Autodesk Inventor part; units mm, degrees
(part 2 of 3)
sketch "Skizze14" plane through (-77, -91.5, 192.5) normal (0.7071, 0, 0.7071) x (0.7071, 0, -0.7071)
  line L0 (0.4493, 19.9089) -> (5.7022, 19.9089) construction
  line L1 (5.7022, 19.9089) -> (5.7022, 29.9599) construction
  line L2 (5.7022, 29.9599) -> (0.4493, 29.9599) construction
  line L3 (0.4493, 29.9599) -> (0.4493, 19.9089) construction
  line L4 (0.4923, 49.8867) -> (5.7451, 49.8867) construction
  line L5 (5.7451, 49.8867) -> (5.7451, 46.2392) construction
  line L6 (5.7451, 46.2392) -> (0.4923, 46.2392) construction
  line L7 (0.4923, 46.2392) -> (0.4923, 49.8867) construction
  line L8 (0.1277, 60.4817) -> (5.3805, 60.4817) construction
  line L9 (5.3805, 60.4817) -> (5.3805, 56.8342) construction
  line L10 (5.3805, 56.8342) -> (0.1277, 56.8342) construction
  line L11 (0.1277, 56.8342) -> (0.1277, 60.4817) construction
  line L12 (0.177, 70.1367) -> (5.4298, 70.1367) construction
  line L13 (5.4298, 70.1367) -> (5.4298, 66.4892) construction
  line L14 (5.4298, 66.4892) -> (0.177, 66.4892) construction
  line L15 (0.177, 66.4892) -> (0.177, 70.1367) construction
  line L16 (0.177, 80.1367) -> (5.4298, 80.1367) construction
  line L17 (5.4298, 80.1367) -> (5.4298, 76.4892) construction
  line L18 (5.4298, 76.4892) -> (0.177, 76.4892) construction
  line L19 (0.177, 76.4892) -> (0.177, 80.1367) construction
  line L20 (0.177, 90.1367) -> (5.4298, 90.1367) construction
  line L21 (5.4298, 90.1367) -> (5.4298, 86.4892) construction
  line L22 (5.4298, 86.4892) -> (0.177, 86.4892) construction
  line L23 (0.177, 86.4892) -> (0.177, 90.1367) construction
  line L24 (0.177, 100.1367) -> (5.4298, 100.1367) construction
  line L25 (5.4298, 100.1367) -> (5.4298, 96.4892) construction
  line L26 (5.4298, 96.4892) -> (0.177, 96.4892) construction
  line L27 (0.177, 96.4892) -> (0.177, 100.1367) construction
  line L28 (0.177, 110.1367) -> (5.4298, 110.1367) construction
  line L29 (5.4298, 110.1367) -> (5.4298, 106.4892) construction
  line L30 (5.4298, 106.4892) -> (0.177, 106.4892) construction
  line L31 (0.177, 106.4892) -> (0.177, 110.1367) construction
  line L32 (-0.2126, 120.6134) -> (5.0402, 120.6134) construction
  line L33 (5.0402, 120.6134) -> (5.0402, 116.9659) construction
  line L34 (5.0402, 116.9659) -> (-0.2126, 116.9659) construction
  line L35 (-0.2126, 116.9659) -> (-0.2126, 120.6134) construction
  line L36 (-0.2161, 130.1063) -> (5.0368, 130.1063) construction
  line L37 (5.0368, 130.1063) -> (5.0368, 126.4588) construction
  line L38 (5.0368, 126.4588) -> (-0.2161, 126.4588) construction
  line L39 (-0.2161, 126.4588) -> (-0.2161, 130.1063) construction
  line L40 (-0.2978, 140.1) -> (4.9551, 140.1) construction
  line L41 (4.9551, 140.1) -> (4.9551, 136.4525) construction
  line L42 (4.9551, 136.4525) -> (-0.2978, 136.4525) construction
  line L43 (-0.2978, 136.4525) -> (-0.2978, 140.1) construction
  line L44 (-0.3019, 150.1519) -> (4.9509, 150.1519) construction
  line L45 (4.9509, 150.1519) -> (4.9509, 146.5044) construction
  line L46 (4.9509, 146.5044) -> (-0.3019, 146.5044) construction
  line L47 (-0.3019, 146.5044) -> (-0.3019, 150.1519) construction
  line L48 (-0.2744, 160.1018) -> (4.9784, 160.1018) construction
  line L49 (4.9784, 160.1018) -> (4.9784, 156.4543) construction
  line L50 (4.9784, 156.4543) -> (-0.2744, 156.4543) construction
  line L51 (-0.2744, 156.4543) -> (-0.2744, 160.1018) construction
  line L52 (-0.539, 170.1317) -> (4.1973, 170.1317) construction
  line L53 (4.1973, 170.1317) -> (4.1973, 166.4842) construction
  line L54 (4.1973, 166.4842) -> (-0.539, 166.4842) construction
  line L55 (-0.539, 166.4842) -> (-0.539, 170.1317) construction
  line L56 (0.5265, 39.54) -> (5.7793, 39.54) construction
  line L57 (5.7793, 39.54) -> (5.7793, 35.8925) construction
  line L58 (5.7793, 35.8925) -> (0.5265, 35.8925) construction
  line L59 (0.5265, 35.8925) -> (0.5265, 39.54) construction
  line L60 (8.4853, 5) -> (8.4853, 29.5) projected
  line L61 (12.1672, 16.75) -> (4.8034, 16.75)
  line L62 (4.8034, 16.75) -> (4.8034, 17.75)
  line L63 (4.8034, 17.75) -> (12.1672, 17.75)
  line L64 (12.1672, 17.75) -> (12.1672, 16.75)
  line L65 (12.1672, 16.75) -> (4.8034, 17.75) construction
  line L66 (4.8034, 16.75) -> (12.1672, 17.75) construction
  line L67 (7.3114, 17.75) -> (7.3114, 16.75)
  line L68 (2.9776, 164.5202) -> (0.2945, 164.5202)
  line L69 (0.2945, 164.5202) -> (0.2945, 165.0818)
  line L70 (0.2945, 165.0818) -> (1.2928, 165.0818)
  line L71 (1.2928, 165.0818) -> (1.2928, 168.7678)
  line L72 (1.2928, 168.7678) -> (0.2945, 168.7678)
  line L73 (0.2945, 168.7678) -> (0.2945, 169.2715)
  spline S0 degree 2 poles (0.2945, 169.2715) (0.8605, 169.2715) (1.3954, 169.5924) (1.431, 170.0381) knots 0 0 0 1 2 2 2
  line L74 (1.431, 170.0381) -> (2.0015, 170.0381)
  line L75 (2.0015, 170.0381) -> (2.0015, 165.0818)
  line L76 (2.0015, 165.0818) -> (2.9776, 165.0818)
  line L77 (2.9776, 165.0818) -> (2.9776, 164.5202)
  spline S1 degree 2 poles (7.4659, 166.3031) (7.4659, 165.8796) (7.1851, 165.1621) (6.9488, 164.9214) knots 0 0 0 1 2 2 2
  spline S2 degree 2 poles (6.9488, 164.9214) (6.7037, 164.6673) (6.0886, 164.4044) (5.7187, 164.4044) knots 0 0 0 1 2 2 2
  spline S3 degree 2 poles (5.7187, 164.4044) (5.3488, 164.4044) (4.7381, 164.6539) (4.5064, 164.9035) knots 0 0 0 1 2 2 2
  spline S4 degree 2 poles (4.5064, 164.9035) (4.2211, 165.2022) (3.9002, 166.205) (3.9002, 166.936) knots 0 0 0 1 2 2 2
  spline S5 degree 2 poles (3.9002, 166.936) (3.9002, 167.6535) (4.1944, 168.8079) (4.5019, 169.2358) knots 0 0 0 1 2 2 2
  spline S6 degree 2 poles (4.5019, 169.2358) (4.8005, 169.6548) (5.7454, 170.1227) (6.365, 170.1227) knots 0 0 0 1 2 2 2
  spline S7 degree 2 poles (6.365, 170.1227) (6.5477, 170.1227) (6.8686, 170.0871) (6.989, 170.047) knots 0 0 0 1 2 2 2
  line L78 (6.989, 170.047) -> (6.989, 169.3383)
  line L79 (6.989, 169.3383) -> (6.9578, 169.3383)
  spline S8 degree 2 poles (6.9578, 169.3383) (6.8552, 169.3918) (6.4808, 169.4854) (6.2669, 169.4854) knots 0 0 0 1 2 2 2
  spline S9 degree 2 poles (6.2669, 169.4854) (5.5805, 169.4854) (4.7381, 168.5583) (4.6579, 167.6491) knots 0 0 0 1 2 2 2
  spline S10 degree 2 poles (4.6579, 167.6491) (4.9209, 167.8318) (5.4736, 168.0324) (5.8034, 168.0324) knots 0 0 0 1 2 2 2
  spline S11 degree 2 poles (5.8034, 168.0324) (6.1243, 168.0324) (6.6056, 167.9031) (6.8686, 167.707) knots 0 0 0 1 2 2 2
  spline S12 degree 2 poles (6.8686, 167.707) (7.1717, 167.4797) (7.4659, 166.7755) (7.4659, 166.3031) knots 0 0 0 1 2 2 2
  spline S13 degree 2 poles (6.7171, 166.2719) (6.7171, 166.6106) (6.5388, 167.0697) (6.3427, 167.2301) knots 0 0 0 1 2 2 2
  spline S14 degree 2 poles (6.3427, 167.2301) (6.1956, 167.346) (5.8301, 167.4218) (5.6385, 167.4218) knots 0 0 0 1 2 2 2
  spline S15 degree 2 poles (5.6385, 167.4218) (5.38, 167.4218) (4.8941, 167.2658) (4.6579, 167.1187) knots 0 0 0 1 2 2 2
  spline S16 degree 2 poles (4.6579, 167.1187) (4.6535, 167.0385) (4.6445, 166.8869) (4.6445, 166.771) knots 0 0 0 1 2 2 2
  spline S17 degree 2 poles (4.6445, 166.771) (4.6445, 166.2005) (4.8674, 165.5008) (5.0368, 165.318) knots 0 0 0 1 2 2 2
  spline S18 degree 2 poles (5.0368, 165.318) (5.1928, 165.1442) (5.5315, 165.0061) (5.7231, 165.0061) knots 0 0 0 1 2 2 2
  spline S19 degree 2 poles (5.7231, 165.0061) (6.1689, 165.0061) (6.7171, 165.639) (6.7171, 166.2719) knots 0 0 0 1 2 2 2
  spline S20 degree 2 poles (11.5396, 167.2702) (11.5396, 165.7905) (10.6794, 164.4044) (9.7835, 164.4044) knots 0 0 0 1 2 2 2
  spline S21 degree 2 poles (9.7835, 164.4044) (8.8743, 164.4044) (8.023, 165.8172) (8.023, 167.2658) knots 0 0 0 1 2 2 2
  spline S22 degree 2 poles (8.023, 167.2658) (8.023, 168.7544) (8.8832, 170.1317) (9.7835, 170.1317) knots 0 0 0 1 2 2 2
  spline S23 degree 2 poles (9.7835, 170.1317) (10.6883, 170.1317) (11.5396, 168.7054) (11.5396, 167.2702) knots 0 0 0 1 2 2 2
  spline S24 degree 2 poles (10.5947, 165.5944) (10.7017, 165.8663) (10.7908, 166.7042) (10.7908, 167.2702) knots 0 0 0 1 2 2 2
  spline S25 degree 2 poles (10.7908, 167.2702) (10.7908, 167.8363) (10.7017, 168.6697) (10.5902, 168.9505) knots 0 0 0 1 2 2 2
  spline S26 degree 2 poles (10.5902, 168.9505) (10.4788, 169.2313) (10.0911, 169.521) (9.7835, 169.521) knots 0 0 0 1 2 2 2
  spline S27 degree 2 poles (9.7835, 169.521) (9.476, 169.521) (9.0793, 169.2313) (8.9634, 168.9416) knots 0 0 0 1 2 2 2
  spline S28 degree 2 poles (8.9634, 168.9416) (8.852, 168.6608) (8.7718, 167.8051) (8.7718, 167.2658) knots 0 0 0 1 2 2 2
  spline S29 degree 2 poles (8.7718, 167.2658) (8.7718, 166.6864) (8.8431, 165.9108) (8.959, 165.6078) knots 0 0 0 1 2 2 2
  spline S30 degree 2 poles (8.959, 165.6078) (9.0659, 165.3225) (9.4626, 165.015) (9.7835, 165.015) knots 0 0 0 1 2 2 2
  spline S31 degree 2 poles (9.7835, 165.015) (10.0866, 165.015) (10.4833, 165.3047) (10.5947, 165.5944) knots 0 0 0 1 2 2 2
  line L80 (3.2422, 154.4903) -> (0.559, 154.4903)
  line L81 (0.559, 154.4903) -> (0.559, 155.0519)
  line L82 (0.559, 155.0519) -> (1.5574, 155.0519)
  line L83 (1.5574, 155.0519) -> (1.5574, 158.7379)
  line L84 (1.5574, 158.7379) -> (0.559, 158.7379)
  line L85 (0.559, 158.7379) -> (0.559, 159.2416)
  spline S32 degree 2 poles (0.559, 159.2416) (1.1251, 159.2416) (1.6599, 159.5625) (1.6956, 160.0082) knots 0 0 0 1 2 2 2
  line L86 (1.6956, 160.0082) -> (2.2661, 160.0082)
  line L87 (2.2661, 160.0082) -> (2.2661, 155.0519)
  line L88 (2.2661, 155.0519) -> (3.2422, 155.0519)
  line L89 (3.2422, 155.0519) -> (3.2422, 154.4903)
  spline S33 degree 2 poles (7.5878, 156.2375) (7.5878, 155.8408) (7.3337, 155.1634) (7.102, 154.9138) knots 0 0 0 1 2 2 2
  spline S34 degree 2 poles (7.102, 154.9138) (6.8702, 154.6642) (6.1794, 154.3745) (5.7515, 154.3745) knots 0 0 0 1 2 2 2
  spline S35 degree 2 poles (5.7515, 154.3745) (5.3593, 154.3745) (4.5927, 154.5483) (4.3119, 154.6865) knots 0 0 0 1 2 2 2
  line L90 (4.3119, 154.6865) -> (4.3119, 155.4664)
  line L91 (4.3119, 155.4664) -> (4.3653, 155.4664)
  spline S36 degree 2 poles (4.3653, 155.4664) (4.45, 155.404) (4.7665, 155.2436) (4.9581, 155.1723) knots 0 0 0 1 2 2 2
  spline S37 degree 2 poles (4.9581, 155.1723) (5.1765, 155.0965) (5.5375, 155.0118) (5.7649, 155.0118) knots 0 0 0 1 2 2 2
  spline S38 degree 2 poles (5.7649, 155.0118) (5.9877, 155.0118) (6.4067, 155.1723) (6.5582, 155.3461) knots 0 0 0 1 2 2 2
  spline S39 degree 2 poles (6.5582, 155.3461) (6.6964, 155.511) (6.839, 155.9478) (6.839, 156.242) knots 0 0 0 1 2 2 2
  spline S40 degree 2 poles (6.839, 156.242) (6.839, 156.5361) (6.6786, 156.9105) (6.527, 157.0353) knots 0 0 0 1 2 2 2
  spline S41 degree 2 poles (6.527, 157.0353) (6.371, 157.1735) (5.9075, 157.2894) (5.6267, 157.2894) knots 0 0 0 1 2 2 2
  spline S42 degree 2 poles (5.6267, 157.2894) (5.3236, 157.2894) (4.7219, 157.1958) (4.5392, 157.1557) knots 0 0 0 1 2 2 2
  line L92 (4.5392, 157.1557) -> (4.5392, 159.9903)
  line L93 (4.5392, 159.9903) -> (7.5566, 159.9903)
  line L94 (7.5566, 159.9903) -> (7.5566, 159.3441)
  line L95 (7.5566, 159.3441) -> (5.2478, 159.3441)
  line L96 (5.2478, 159.3441) -> (5.2478, 157.8777)
  spline S43 degree 2 poles (5.2478, 157.8777) (5.3816, 157.8955) (5.6401, 157.9089) (5.747, 157.9089) knots 0 0 0 1 2 2 2
  spline S44 degree 2 poles (5.747, 157.9089) (6.1705, 157.9089) (6.7543, 157.7707) (7.0217, 157.5657) knots 0 0 0 1 2 2 2
  spline S45 degree 2 poles (7.0217, 157.5657) (7.2936, 157.3607) (7.5878, 156.7367) (7.5878, 156.2375) knots 0 0 0 1 2 2 2
  spline S46 degree 2 poles (11.8042, 157.2403) (11.8042, 155.7606) (10.944, 154.3745) (10.0481, 154.3745) knots 0 0 0 1 2 2 2
  spline S47 degree 2 poles (10.0481, 154.3745) (9.1388, 154.3745) (8.2875, 155.7874) (8.2875, 157.2359) knots 0 0 0 1 2 2 2
  spline S48 degree 2 poles (8.2875, 157.2359) (8.2875, 158.7245) (9.1478, 160.1018) (10.0481, 160.1018) knots 0 0 0 1 2 2 2
  spline S49 degree 2 poles (10.0481, 160.1018) (10.9529, 160.1018) (11.8042, 158.6755) (11.8042, 157.2403) knots 0 0 0 1 2 2 2
  spline S50 degree 2 poles (10.8593, 155.5645) (10.9662, 155.8364) (11.0554, 156.6743) (11.0554, 157.2403) knots 0 0 0 1 2 2 2
  spline S51 degree 2 poles (11.0554, 157.2403) (11.0554, 157.8064) (10.9662, 158.6399) (10.8548, 158.9207) knots 0 0 0 1 2 2 2
  spline S52 degree 2 poles (10.8548, 158.9207) (10.7434, 159.2015) (10.3556, 159.4912) (10.0481, 159.4912) knots 0 0 0 1 2 2 2
  spline S53 degree 2 poles (10.0481, 159.4912) (9.7405, 159.4912) (9.3439, 159.2015) (9.228, 158.9117) knots 0 0 0 1 2 2 2
  spline S54 degree 2 poles (9.228, 158.9117) (9.1166, 158.6309) (9.0363, 157.7752) (9.0363, 157.2359) knots 0 0 0 1 2 2 2
  spline S55 degree 2 poles (9.0363, 157.2359) (9.0363, 156.6565) (9.1076, 155.8809) (9.2235, 155.5779) knots 0 0 0 1 2 2 2
  spline S56 degree 2 poles (9.2235, 155.5779) (9.3305, 155.2926) (9.7272, 154.9851) (10.0481, 154.9851) knots 0 0 0 1 2 2 2
  spline S57 degree 2 poles (10.0481, 154.9851) (10.3512, 154.9851) (10.7478, 155.2748) (10.8593, 155.5645) knots 0 0 0 1 2 2 2
  line L97 (3.2147, 144.536) -> (0.5316, 144.536)
  line L98 (0.5316, 144.536) -> (0.5316, 145.0976)
  line L99 (0.5316, 145.0976) -> (1.53, 145.0976)
  line L100 (1.53, 145.0976) -> (1.53, 148.7836)
  line L101 (1.53, 148.7836) -> (0.5316, 148.7836)
  line L102 (0.5316, 148.7836) -> (0.5316, 149.2872)
  spline S58 degree 2 poles (0.5316, 149.2872) (1.0976, 149.2872) (1.6325, 149.6081) (1.6681, 150.0538) knots 0 0 0 1 2 2 2
  line L103 (1.6681, 150.0538) -> (2.2386, 150.0538)
  line L104 (2.2386, 150.0538) -> (2.2386, 145.0976)
  line L105 (2.2386, 145.0976) -> (3.2147, 145.0976)
  line L106 (3.2147, 145.0976) -> (3.2147, 144.536)
  spline S59 degree 2 poles (5.7107, 149.5145) (5.5101, 149.5145) (5.1134, 149.4165) (4.9218, 149.3407) knots 0 0 0 1 2 2 2
  spline S60 degree 2 poles (4.9218, 149.3407) (4.7435, 149.2649) (4.4805, 149.1045) (4.378, 149.0332) knots 0 0 0 1 2 2 2
  line L107 (4.378, 149.0332) -> (4.3334, 149.0332)
  line L108 (4.3334, 149.0332) -> (4.3334, 149.8132)
  spline S61 degree 2 poles (4.3334, 149.8132) (4.5741, 149.9424) (5.3987, 150.1519) (5.7686, 150.1519) knots 0 0 0 1 2 2 2
  spline S62 degree 2 poles (5.7686, 150.1519) (6.143, 150.1519) (6.7001, 150.0004) (6.9274, 149.8399) knots 0 0 0 1 2 2 2
  spline S63 degree 2 poles (6.9274, 149.8399) (7.1681, 149.6661) (7.4177, 149.1624) (7.4177, 148.8237) knots 0 0 0 1 2 2 2
  spline S64 degree 2 poles (7.4177, 148.8237) (7.4177, 148.3691) (6.8205, 147.6827) (6.4015, 147.5935) knots 0 0 0 1 2 2 2
  line L109 (6.4015, 147.5935) -> (6.4015, 147.5401)
  spline S65 degree 2 poles (6.4015, 147.5401) (6.5753, 147.5044) (6.972, 147.344) (7.1414, 147.1835) knots 0 0 0 1 2 2 2
  spline S66 degree 2 poles (7.1414, 147.1835) (7.3107, 147.0275) (7.5247, 146.5283) (7.5247, 146.1673) knots 0 0 0 1 2 2 2
  spline S67 degree 2 poles (7.5247, 146.1673) (7.5247, 145.7974) (7.2706, 145.1689) (7.0389, 144.9282) knots 0 0 0 1 2 2 2
  spline S68 degree 2 poles (7.0389, 144.9282) (6.7982, 144.6786) (6.1163, 144.4201) (5.6839, 144.4201) knots 0 0 0 1 2 2 2
  spline S69 degree 2 poles (5.6839, 144.4201) (5.2694, 144.4201) (4.4582, 144.6207) (4.1819, 144.7589) knots 0 0 0 1 2 2 2
  line L110 (4.1819, 144.7589) -> (4.1819, 145.5388)
  line L111 (4.1819, 145.5388) -> (4.2354, 145.5388)
  spline S70 degree 2 poles (4.2354, 145.5388) (4.4671, 145.3695) (5.2516, 145.0575) (5.6394, 145.0575) knots 0 0 0 1 2 2 2
  spline S71 degree 2 poles (5.6394, 145.0575) (5.8667, 145.0575) (6.3213, 145.2001) (6.4728, 145.365) knots 0 0 0 1 2 2 2
  spline S72 degree 2 poles (6.4728, 145.365) (6.6199, 145.5299) (6.7759, 145.9222) (6.7759, 146.2208) knots 0 0 0 1 2 2 2
  spline S73 degree 2 poles (6.7759, 146.2208) (6.7759, 146.5194) (6.6021, 146.9072) (6.4461, 147.0186) knots 0 0 0 1 2 2 2
  spline S74 degree 2 poles (6.4461, 147.0186) (6.2901, 147.13) (5.8667, 147.2147) (5.6171, 147.2147) knots 0 0 0 1 2 2 2
  line L112 (5.6171, 147.2147) -> (5.3051, 147.2147)
  line L113 (5.3051, 147.2147) -> (5.3051, 147.8253)
  line L114 (5.3051, 147.8253) -> (5.5502, 147.8253)
  spline S75 degree 2 poles (5.5502, 147.8253) (6.0449, 147.8253) (6.6689, 148.2978) (6.6689, 148.7479) knots 0 0 0 1 2 2 2
  spline S76 degree 2 poles (6.6689, 148.7479) (6.6689, 148.9574) (6.5085, 149.256) (6.3792, 149.3452) knots 0 0 0 1 2 2 2
  spline S77 degree 2 poles (6.3792, 149.3452) (6.2411, 149.4388) (5.9023, 149.5145) (5.7107, 149.5145) knots 0 0 0 1 2 2 2
  spline S78 degree 2 poles (11.7767, 147.286) (11.7767, 145.8063) (10.9165, 144.4201) (10.0206, 144.4201) knots 0 0 0 1 2 2 2
  spline S79 degree 2 poles (10.0206, 144.4201) (9.1114, 144.4201) (8.2601, 145.833) (8.2601, 147.2816) knots 0 0 0 1 2 2 2
  spline S80 degree 2 poles (8.2601, 147.2816) (8.2601, 148.7702) (9.1203, 150.1474) (10.0206, 150.1474) knots 0 0 0 1 2 2 2
  spline S81 degree 2 poles (10.0206, 150.1474) (10.9254, 150.1474) (11.7767, 148.7212) (11.7767, 147.286) knots 0 0 0 1 2 2 2
  spline S82 degree 2 poles (10.8318, 145.6102) (10.9388, 145.882) (11.0279, 146.72) (11.0279, 147.286) knots 0 0 0 1 2 2 2
  spline S83 degree 2 poles (11.0279, 147.286) (11.0279, 147.8521) (10.9388, 148.6855) (10.8274, 148.9663) knots 0 0 0 1 2 2 2
  spline S84 degree 2 poles (10.8274, 148.9663) (10.7159, 149.2471) (10.3282, 149.5368) (10.0206, 149.5368) knots 0 0 0 1 2 2 2
  spline S85 degree 2 poles (10.0206, 149.5368) (9.7131, 149.5368) (9.3164, 149.2471) (9.2005, 148.9574) knots 0 0 0 1 2 2 2
  spline S86 degree 2 poles (9.2005, 148.9574) (9.0891, 148.6766) (9.0089, 147.8209) (9.0089, 147.2816) knots 0 0 0 1 2 2 2
  spline S87 degree 2 poles (9.0089, 147.2816) (9.0089, 146.7021) (9.0802, 145.9266) (9.1961, 145.6235) knots 0 0 0 1 2 2 2
  spline S88 degree 2 poles (9.1961, 145.6235) (9.303, 145.3383) (9.6997, 145.0307) (10.0206, 145.0307) knots 0 0 0 1 2 2 2
  spline S89 degree 2 poles (10.0206, 145.0307) (10.3237, 145.0307) (10.7204, 145.3205) (10.8318, 145.6102) knots 0 0 0 1 2 2 2
  line L115 (3.2189, 134.4841) -> (0.5357, 134.4841)
  line L116 (0.5357, 134.4841) -> (0.5357, 135.0457)
  line L117 (0.5357, 135.0457) -> (1.5341, 135.0457)
  line L118 (1.5341, 135.0457) -> (1.5341, 138.7317)
  line L119 (1.5341, 138.7317) -> (0.5357, 138.7317)
  line L120 (0.5357, 138.7317) -> (0.5357, 139.2353)
  spline S90 degree 2 poles (0.5357, 139.2353) (1.1018, 139.2353) (1.6366, 139.5562) (1.6723, 140.0019) knots 0 0 0 1 2 2 2
  line L121 (1.6723, 140.0019) -> (2.2428, 140.0019)
  line L122 (2.2428, 140.0019) -> (2.2428, 135.0457)
  line L123 (2.2428, 135.0457) -> (3.2189, 135.0457)
  line L124 (3.2189, 135.0457) -> (3.2189, 134.4841)
  line L125 (7.6224, 134.4841) -> (4.2306, 134.4841)
  line L126 (4.2306, 134.4841) -> (4.2306, 135.2641)
  spline S91 degree 2 poles (4.2306, 135.2641) (4.5961, 135.6073) (5.2468, 136.2446) (5.5588, 136.5878) knots 0 0 0 1 2 2 2
  spline S92 degree 2 poles (5.5588, 136.5878) (6.1872, 137.2787) (6.6463, 138.1077) (6.6463, 138.5489) knots 0 0 0 1 2 2 2
  spline S93 degree 2 poles (6.6463, 138.5489) (6.6463, 138.7807) (6.5037, 139.1283) (6.3744, 139.2398) knots 0 0 0 1 2 2 2
  spline S94 degree 2 poles (6.3744, 139.2398) (6.2452, 139.3512) (5.9065, 139.4626) (5.7014, 139.4626) knots 0 0 0 1 2 2 2
  spline S95 degree 2 poles (5.7014, 139.4626) (5.5053, 139.4626) (5.1042, 139.3646) (4.9214, 139.2888) knots 0 0 0 1 2 2 2
  spline S96 degree 2 poles (4.9214, 139.2888) (4.7654, 139.2264) (4.4757, 139.0481) (4.3866, 138.9857) knots 0 0 0 1 2 2 2
  line L127 (4.3866, 138.9857) -> (4.3465, 138.9857)
  line L128 (4.3465, 138.9857) -> (4.3465, 139.7701)
  spline S97 degree 2 poles (4.3465, 139.7701) (4.5738, 139.8816) (5.3894, 140.1) (5.7549, 140.1) knots 0 0 0 1 2 2 2
  spline S98 degree 2 poles (5.7549, 140.1) (6.526, 140.1) (7.3951, 139.2843) (7.3951, 138.589) knots 0 0 0 1 2 2 2
  spline S99 degree 2 poles (7.3951, 138.589) (7.3951, 138.2637) (7.2436, 137.7199) (7.1099, 137.4881) knots 0 0 0 1 2 2 2
  spline S100 degree 2 poles (7.1099, 137.4881) (6.9761, 137.2475) (6.5884, 136.775) (6.3744, 136.5477) knots 0 0 0 1 2 2 2
  spline S101 degree 2 poles (6.3744, 136.5477) (6.0268, 136.1689) (5.1755, 135.3577) (4.9214, 135.1214) knots 0 0 0 1 2 2 2
  line L129 (4.9214, 135.1214) -> (7.6224, 135.1214)
  line L130 (7.6224, 135.1214) -> (7.6224, 134.4841)
  spline S102 degree 2 poles (11.7808, 137.2341) (11.7808, 135.7543) (10.9206, 134.3682) (10.0248, 134.3682) knots 0 0 0 1 2 2 2
  spline S103 degree 2 poles (10.0248, 134.3682) (9.1155, 134.3682) (8.2642, 135.7811) (8.2642, 137.2296) knots 0 0 0 1 2 2 2
  spline S104 degree 2 poles (8.2642, 137.2296) (8.2642, 138.7183) (9.1244, 140.0955) (10.0248, 140.0955) knots 0 0 0 1 2 2 2
  spline S105 degree 2 poles (10.0248, 140.0955) (10.9295, 140.0955) (11.7808, 138.6693) (11.7808, 137.2341) knots 0 0 0 1 2 2 2
  spline S106 degree 2 poles (10.836, 135.5582) (10.9429, 135.8301) (11.0321, 136.668) (11.0321, 137.2341) knots 0 0 0 1 2 2 2
  spline S107 degree 2 poles (11.0321, 137.2341) (11.0321, 137.8001) (10.9429, 138.6336) (10.8315, 138.9144) knots 0 0 0 1 2 2 2
  spline S108 degree 2 poles (10.8315, 138.9144) (10.7201, 139.1952) (10.3323, 139.4849) (10.0248, 139.4849) knots 0 0 0 1 2 2 2
  spline S109 degree 2 poles (10.0248, 139.4849) (9.7172, 139.4849) (9.3206, 139.1952) (9.2047, 138.9055) knots 0 0 0 1 2 2 2
  spline S110 degree 2 poles (9.2047, 138.9055) (9.0932, 138.6247) (9.013, 137.7689) (9.013, 137.2296) knots 0 0 0 1 2 2 2
  spline S111 degree 2 poles (9.013, 137.2296) (9.013, 136.6502) (9.0843, 135.8747) (9.2002, 135.5716) knots 0 0 0 1 2 2 2
  spline S112 degree 2 poles (9.2002, 135.5716) (9.3072, 135.2864) (9.7039, 134.9788) (10.0248, 134.9788) knots 0 0 0 1 2 2 2
  spline S113 degree 2 poles (10.0248, 134.9788) (10.3278, 134.9788) (10.7245, 135.2685) (10.836, 135.5582) knots 0 0 0 1 2 2 2
  line L131 (3.3005, 124.4949) -> (0.6174, 124.4949)
  line L132 (0.6174, 124.4949) -> (0.6174, 125.0565)
  line L133 (0.6174, 125.0565) -> (1.6158, 125.0565)
  line L134 (1.6158, 125.0565) -> (1.6158, 128.7424)
  line L135 (1.6158, 128.7424) -> (0.6174, 128.7424)
  line L136 (0.6174, 128.7424) -> (0.6174, 129.2461)
  spline S114 degree 2 poles (0.6174, 129.2461) (1.1834, 129.2461) (1.7183, 129.567) (1.754, 130.0127) knots 0 0 0 1 2 2 2
  line L137 (1.754, 130.0127) -> (2.3245, 130.0127)
  line L138 (2.3245, 130.0127) -> (2.3245, 125.0565)
  line L139 (2.3245, 125.0565) -> (3.3005, 125.0565)
  line L140 (3.3005, 125.0565) -> (3.3005, 124.4949)
  line L141 (7.4278, 124.4949) -> (4.7446, 124.4949)
  line L142 (4.7446, 124.4949) -> (4.7446, 125.0565)
  line L143 (4.7446, 125.0565) -> (5.743, 125.0565)
  line L144 (5.743, 125.0565) -> (5.743, 128.7424)
  line L145 (5.743, 128.7424) -> (4.7446, 128.7424)
  line L146 (4.7446, 128.7424) -> (4.7446, 129.2461)
  spline S115 degree 2 poles (4.7446, 129.2461) (5.3107, 129.2461) (5.8455, 129.567) (5.8812, 130.0127) knots 0 0 0 1 2 2 2
  line L147 (5.8812, 130.0127) -> (6.4517, 130.0127)
  line L148 (6.4517, 130.0127) -> (6.4517, 125.0565)
  line L149 (6.4517, 125.0565) -> (7.4278, 125.0565)
  line L150 (7.4278, 125.0565) -> (7.4278, 124.4949)
  spline S116 degree 2 poles (11.8625, 127.2449) (11.8625, 125.7651) (11.0023, 124.379) (10.1065, 124.379) knots 0 0 0 1 2 2 2
  spline S117 degree 2 poles (10.1065, 124.379) (9.1972, 124.379) (8.3459, 125.7919) (8.3459, 127.2404) knots 0 0 0 1 2 2 2
  spline S118 degree 2 poles (8.3459, 127.2404) (8.3459, 128.7291) (9.2061, 130.1063) (10.1065, 130.1063) knots 0 0 0 1 2 2 2
  spline S119 degree 2 poles (10.1065, 130.1063) (11.0112, 130.1063) (11.8625, 128.68) (11.8625, 127.2449) knots 0 0 0 1 2 2 2
  spline S120 degree 2 poles (10.9176, 125.569) (11.0246, 125.8409) (11.1138, 126.6788) (11.1138, 127.2449) knots 0 0 0 1 2 2 2
  spline S121 degree 2 poles (11.1138, 127.2449) (11.1138, 127.8109) (11.0246, 128.6444) (10.9132, 128.9252) knots 0 0 0 1 2 2 2
  spline S122 degree 2 poles (10.9132, 128.9252) (10.8018, 129.206) (10.414, 129.4957) (10.1065, 129.4957) knots 0 0 0 1 2 2 2
  spline S123 degree 2 poles (10.1065, 129.4957) (9.7989, 129.4957) (9.4022, 129.206) (9.2864, 128.9163) knots 0 0 0 1 2 2 2
  spline S124 degree 2 poles (9.2864, 128.9163) (9.1749, 128.6355) (9.0947, 127.7797) (9.0947, 127.2404) knots 0 0 0 1 2 2 2
  spline S125 degree 2 poles (9.0947, 127.2404) (9.0947, 126.661) (9.166, 125.8855) (9.2819, 125.5824) knots 0 0 0 1 2 2 2
  spline S126 degree 2 poles (9.2819, 125.5824) (9.3889, 125.2971) (9.7856, 124.9896) (10.1065, 124.9896) knots 0 0 0 1 2 2 2
  spline S127 degree 2 poles (10.1065, 124.9896) (10.4095, 124.9896) (10.8062, 125.2793) (10.9176, 125.569) knots 0 0 0 1 2 2 2
  line L151 (3.304, 115.002) -> (0.6208, 115.002)
  line L152 (0.6208, 115.002) -> (0.6208, 115.5635)
  line L153 (0.6208, 115.5635) -> (1.6192, 115.5635)
  line L154 (1.6192, 115.5635) -> (1.6192, 119.2495)
  line L155 (1.6192, 119.2495) -> (0.6208, 119.2495)
  line L156 (0.6208, 119.2495) -> (0.6208, 119.7532)
  spline S128 degree 2 poles (0.6208, 119.7532) (1.1869, 119.7532) (1.7217, 120.0741) (1.7574, 120.5198) knots 0 0 0 1 2 2 2
  line L157 (1.7574, 120.5198) -> (2.3279, 120.5198)
  line L158 (2.3279, 120.5198) -> (2.3279, 115.5635)
  line L159 (2.3279, 115.5635) -> (3.304, 115.5635)
  line L160 (3.304, 115.5635) -> (3.304, 115.002)
  spline S129 degree 2 poles (7.7387, 117.752) (7.7387, 116.2722) (6.8785, 114.8861) (5.9827, 114.8861) knots 0 0 0 1 2 2 2
  spline S130 degree 2 poles (5.9827, 114.8861) (5.0734, 114.8861) (4.2221, 116.299) (4.2221, 117.7475) knots 0 0 0 1 2 2 2
  spline S131 degree 2 poles (4.2221, 117.7475) (4.2221, 119.2362) (5.0823, 120.6134) (5.9827, 120.6134) knots 0 0 0 1 2 2 2
  spline S132 degree 2 poles (5.9827, 120.6134) (6.8874, 120.6134) (7.7387, 119.1871) (7.7387, 117.752) knots 0 0 0 1 2 2 2
  spline S133 degree 2 poles (6.7938, 116.0761) (6.9008, 116.348) (6.99, 117.1859) (6.99, 117.752) knots 0 0 0 1 2 2 2
  spline S134 degree 2 poles (6.99, 117.752) (6.99, 118.318) (6.9008, 119.1515) (6.7894, 119.4323) knots 0 0 0 1 2 2 2
  spline S135 degree 2 poles (6.7894, 119.4323) (6.678, 119.7131) (6.2902, 120.0028) (5.9827, 120.0028) knots 0 0 0 1 2 2 2
  spline S136 degree 2 poles (5.9827, 120.0028) (5.6751, 120.0028) (5.2784, 119.7131) (5.1626, 119.4233) knots 0 0 0 1 2 2 2
  spline S137 degree 2 poles (5.1626, 119.4233) (5.0511, 119.1426) (4.9709, 118.2868) (4.9709, 117.7475) knots 0 0 0 1 2 2 2
  spline S138 degree 2 poles (4.9709, 117.7475) (4.9709, 117.1681) (5.0422, 116.3926) (5.1581, 116.0895) knots 0 0 0 1 2 2 2
  spline S139 degree 2 poles (5.1581, 116.0895) (5.2651, 115.8042) (5.6617, 115.4967) (5.9827, 115.4967) knots 0 0 0 1 2 2 2
  spline S140 degree 2 poles (5.9827, 115.4967) (6.2857, 115.4967) (6.6824, 115.7864) (6.7938, 116.0761) knots 0 0 0 1 2 2 2
  spline S141 degree 2 poles (11.866, 117.752) (11.866, 116.2722) (11.0058, 114.8861) (10.1099, 114.8861) knots 0 0 0 1 2 2 2
  spline S142 degree 2 poles (10.1099, 114.8861) (9.2006, 114.8861) (8.3494, 116.299) (8.3494, 117.7475) knots 0 0 0 1 2 2 2
  spline S143 degree 2 poles (8.3494, 117.7475) (8.3494, 119.2362) (9.2096, 120.6134) (10.1099, 120.6134) knots 0 0 0 1 2 2 2
  spline S144 degree 2 poles (10.1099, 120.6134) (11.0147, 120.6134) (11.866, 119.1871) (11.866, 117.752) knots 0 0 0 1 2 2 2
  spline S145 degree 2 poles (10.9211, 116.0761) (11.028, 116.348) (11.1172, 117.1859) (11.1172, 117.752) knots 0 0 0 1 2 2 2
  spline S146 degree 2 poles (11.1172, 117.752) (11.1172, 118.318) (11.028, 119.1515) (10.9166, 119.4323) knots 0 0 0 1 2 2 2
  spline S147 degree 2 poles (10.9166, 119.4323) (10.8052, 119.7131) (10.4174, 120.0028) (10.1099, 120.0028) knots 0 0 0 1 2 2 2
  spline S148 degree 2 poles (10.1099, 120.0028) (9.8023, 120.0028) (9.4057, 119.7131) (9.2898, 119.4233) knots 0 0 0 1 2 2 2
  spline S149 degree 2 poles (9.2898, 119.4233) (9.1784, 119.1426) (9.0981, 118.2868) (9.0981, 117.7475) knots 0 0 0 1 2 2 2
  spline S150 degree 2 poles (9.0981, 117.7475) (9.0981, 117.1681) (9.1694, 116.3926) (9.2853, 116.0895) knots 0 0 0 1 2 2 2
  spline S151 degree 2 poles (9.2853, 116.0895) (9.3923, 115.8042) (9.789, 115.4967) (10.1099, 115.4967) knots 0 0 0 1 2 2 2
  spline S152 degree 2 poles (10.1099, 115.4967) (10.413, 115.4967) (10.8096, 115.7864) (10.9211, 116.0761) knots 0 0 0 1 2 2 2
  spline S153 degree 2 poles (0.4266, 108.238) (0.4266, 108.6614) (0.7029, 109.3657) (0.9436, 109.6197) knots 0 0 0 1 2 2 2
  spline S154 degree 2 poles (0.9436, 109.6197) (1.1709, 109.8648) (1.835, 110.1367) (2.1737, 110.1367) knots 0 0 0 1 2 2 2
  spline S155 degree 2 poles (2.1737, 110.1367) (2.5526, 110.1367) (3.1676, 109.8827) (3.395, 109.642) knots 0 0 0 1 2 2 2
  spline S156 degree 2 poles (3.395, 109.642) (3.6802, 109.3389) (3.9922, 108.3584) (3.9922, 107.6051) knots 0 0 0 1 2 2 2
  spline S157 degree 2 poles (3.9922, 107.6051) (3.9922, 106.9232) (3.6847, 105.702) (3.386, 105.2964) knots 0 0 0 1 2 2 2
  spline S158 degree 2 poles (3.386, 105.2964) (3.0696, 104.8685) (2.1782, 104.4183) (1.5275, 104.4183) knots 0 0 0 1 2 2 2
  spline S159 degree 2 poles (1.5275, 104.4183) (1.3804, 104.4183) (1.0461, 104.4495) (0.9035, 104.4941) knots 0 0 0 1 2 2 2
  line L161 (0.9035, 104.4941) -> (0.9035, 105.2028)
  line L162 (0.9035, 105.2028) -> (0.9391, 105.2028)
  spline S160 degree 2 poles (0.9391, 105.2028) (1.0327, 105.1493) (1.4249, 105.0557) (1.6255, 105.0557) knots 0 0 0 1 2 2 2
  spline S161 degree 2 poles (1.6255, 105.0557) (2.3475, 105.0557) (3.1721, 106.0095) (3.23, 106.892) knots 0 0 0 1 2 2 2
  spline S162 degree 2 poles (3.23, 106.892) (2.9359, 106.6914) (2.401, 106.5087) (2.0846, 106.5087) knots 0 0 0 1 2 2 2
  spline S163 degree 2 poles (2.0846, 106.5087) (1.7815, 106.5087) (1.2779, 106.6424) (1.0238, 106.8341) knots 0 0 0 1 2 2 2
  spline S164 degree 2 poles (1.0238, 106.8341) (0.7296, 107.0614) (0.4266, 107.7522) (0.4266, 108.238) knots 0 0 0 1 2 2 2
  spline S165 degree 2 poles (3.2479, 107.77) (3.2479, 108.3272) (3.0428, 109.0314) (2.8601, 109.223) knots 0 0 0 1 2 2 2
  spline S166 degree 2 poles (2.8601, 109.223) (2.6997, 109.4013) (2.3654, 109.535) (2.1693, 109.535) knots 0 0 0 1 2 2 2
  spline S167 degree 2 poles (2.1693, 109.535) (1.7146, 109.535) (1.1753, 108.8843) (1.1753, 108.2692) knots 0 0 0 1 2 2 2
  spline S168 degree 2 poles (1.1753, 108.2692) (1.1753, 107.9216) (1.3536, 107.4714) (1.5497, 107.311) knots 0 0 0 1 2 2 2
  spline S169 degree 2 poles (1.5497, 107.311) (1.6924, 107.1951) (2.0445, 107.1193) (2.2495, 107.1193) knots 0 0 0 1 2 2 2
  spline S170 degree 2 poles (2.2495, 107.1193) (2.4857, 107.1193) (3.0295, 107.2842) (3.2345, 107.4224) knots 0 0 0 1 2 2 2
  spline S171 degree 2 poles (3.2345, 107.4224) (3.239, 107.4759) (3.2479, 107.6586) (3.2479, 107.77) knots 0 0 0 1 2 2 2
  spline S172 degree 2 poles (8.1283, 107.2753) (8.1283, 105.7956) (7.2681, 104.4094) (6.3723, 104.4094) knots 0 0 0 1 2 2 2
  spline S173 degree 2 poles (6.3723, 104.4094) (5.463, 104.4094) (4.6117, 105.8223) (4.6117, 107.2708) knots 0 0 0 1 2 2 2
  spline S174 degree 2 poles (4.6117, 107.2708) (4.6117, 108.7595) (5.4719, 110.1367) (6.3723, 110.1367) knots 0 0 0 1 2 2 2
  spline S175 degree 2 poles (6.3723, 110.1367) (7.277, 110.1367) (8.1283, 108.7105) (8.1283, 107.2753) knots 0 0 0 1 2 2 2
  spline S176 degree 2 poles (7.1834, 105.5994) (7.2904, 105.8713) (7.3796, 106.7093) (7.3796, 107.2753) knots 0 0 0 1 2 2 2
  spline S177 degree 2 poles (7.3796, 107.2753) (7.3796, 107.8413) (7.2904, 108.6748) (7.179, 108.9556) knots 0 0 0 1 2 2 2
  spline S178 degree 2 poles (7.179, 108.9556) (7.0676, 109.2364) (6.6798, 109.5261) (6.3723, 109.5261) knots 0 0 0 1 2 2 2
  spline S179 degree 2 poles (6.3723, 109.5261) (6.0647, 109.5261) (5.6681, 109.2364) (5.5522, 108.9467) knots 0 0 0 1 2 2 2
  spline S180 degree 2 poles (5.5522, 108.9467) (5.4407, 108.6659) (5.3605, 107.8101) (5.3605, 107.2708) knots 0 0 0 1 2 2 2
  spline S181 degree 2 poles (5.3605, 107.2708) (5.3605, 106.6914) (5.4318, 105.9159) (5.5477, 105.6128) knots 0 0 0 1 2 2 2
  spline S182 degree 2 poles (5.5477, 105.6128) (5.6547, 105.3276) (6.0514, 105.02) (6.3723, 105.02) knots 0 0 0 1 2 2 2
  spline S183 degree 2 poles (6.3723, 105.02) (6.6753, 105.02) (7.072, 105.3097) (7.1834, 105.5994) knots 0 0 0 1 2 2 2
  spline S184 degree 2 poles (2.2406, 94.3871) (1.8305, 94.3871) (1.1575, 94.6323) (0.9213, 94.8596) knots 0 0 0 1 2 2 2
  spline S185 degree 2 poles (0.9213, 94.8596) (0.6895, 95.0824) (0.4488, 95.6886) (0.4488, 96.0318) knots 0 0 0 1 2 2 2
  spline S186 degree 2 poles (0.4488, 96.0318) (0.4488, 96.4775) (0.9257, 97.2263) (1.3804, 97.4491) knots 0 0 0 1 2 2 2
  line L163 (1.3804, 97.4491) -> (1.3804, 97.4714)
  spline S187 degree 2 poles (1.3804, 97.4714) (0.9748, 97.7076) (0.5826, 98.2692) (0.5826, 98.6882) knots 0 0 0 1 2 2 2
  spline S188 degree 2 poles (0.5826, 98.6882) (0.5826, 99.3077) (1.5185, 100.1367) (2.2406, 100.1367) knots 0 0 0 1 2 2 2
  spline S189 degree 2 poles (2.2406, 100.1367) (2.9894, 100.1367) (3.8941, 99.3523) (3.8941, 98.7372) knots 0 0 0 1 2 2 2
  spline S190 degree 2 poles (3.8941, 98.7372) (3.8941, 98.3673) (3.4618, 97.6452) (3.0562, 97.4402) knots 0 0 0 1 2 2 2
  line L164 (3.0562, 97.4402) -> (3.0562, 97.4179)
  spline S191 degree 2 poles (3.0562, 97.4179) (3.5376, 97.1951) (4.0323, 96.5533) (4.0323, 96.0452) knots 0 0 0 1 2 2 2
  spline S192 degree 2 poles (4.0323, 96.0452) (4.0323, 95.3409) (3.0072, 94.3871) (2.2406, 94.3871) knots 0 0 0 1 2 2 2
  spline S193 degree 2 poles (3.2746, 95.9738) (3.2746, 96.3126) (3.0072, 96.7137) (2.6283, 96.9187) knots 0 0 0 1 2 2 2
  spline S194 degree 2 poles (2.6283, 96.9187) (2.5035, 96.99) (2.0846, 97.155) (1.8216, 97.2619) knots 0 0 0 1 2 2 2
  spline S195 degree 2 poles (1.8216, 97.2619) (1.5185, 97.0614) (1.1932, 96.4641) (1.1932, 96.0853) knots 0 0 0 1 2 2 2
  spline S196 degree 2 poles (1.1932, 96.0853) (1.1932, 95.5861) (1.7949, 94.9353) (2.2495, 94.9353) knots 0 0 0 1 2 2 2
  spline S197 degree 2 poles (2.2495, 94.9353) (2.713, 94.9353) (3.2746, 95.4925) (3.2746, 95.9738) knots 0 0 0 1 2 2 2
  spline S198 degree 2 poles (3.1721, 98.7283) (3.1721, 99.0982) (2.6774, 99.593) (2.2361, 99.593) knots 0 0 0 1 2 2 2
  spline S199 degree 2 poles (2.2361, 99.593) (1.835, 99.593) (1.3224, 99.1517) (1.3224, 98.7729) knots 0 0 0 1 2 2 2
  spline S200 degree 2 poles (1.3224, 98.7729) (1.3224, 98.501) (1.5854, 98.1221) (1.8484, 97.9706) knots 0 0 0 1 2 2 2
  spline S201 degree 2 poles (1.8484, 97.9706) (1.9598, 97.9082) (2.4322, 97.6898) (2.6239, 97.6274) knots 0 0 0 1 2 2 2
  spline S202 degree 2 poles (2.6239, 97.6274) (2.9448, 97.8725) (3.1721, 98.394) (3.1721, 98.7283) knots 0 0 0 1 2 2 2
  spline S203 degree 2 poles (8.1283, 97.2619) (8.1283, 95.7822) (7.2681, 94.396) (6.3723, 94.396) knots 0 0 0 1 2 2 2
  spline S204 degree 2 poles (6.3723, 94.396) (5.463, 94.396) (4.6117, 95.8089) (4.6117, 97.2575) knots 0 0 0 1 2 2 2
  spline S205 degree 2 poles (4.6117, 97.2575) (4.6117, 98.7461) (5.4719, 100.1234) (6.3723, 100.1234) knots 0 0 0 1 2 2 2
  spline S206 degree 2 poles (6.3723, 100.1234) (7.277, 100.1234) (8.1283, 98.6971) (8.1283, 97.2619) knots 0 0 0 1 2 2 2
  spline S207 degree 2 poles (7.1834, 95.5861) (7.2904, 95.858) (7.3796, 96.6959) (7.3796, 97.2619) knots 0 0 0 1 2 2 2
  spline S208 degree 2 poles (7.3796, 97.2619) (7.3796, 97.828) (7.2904, 98.6614) (7.179, 98.9422) knots 0 0 0 1 2 2 2
  spline S209 degree 2 poles (7.179, 98.9422) (7.0676, 99.223) (6.6798, 99.5127) (6.3723, 99.5127) knots 0 0 0 1 2 2 2
  spline S210 degree 2 poles (6.3723, 99.5127) (6.0647, 99.5127) (5.6681, 99.223) (5.5522, 98.9333) knots 0 0 0 1 2 2 2
  spline S211 degree 2 poles (5.5522, 98.9333) (5.4407, 98.6525) (5.3605, 97.7968) (5.3605, 97.2575) knots 0 0 0 1 2 2 2
  spline S212 degree 2 poles (5.3605, 97.2575) (5.3605, 96.6781) (5.4318, 95.9025) (5.5477, 95.5994) knots 0 0 0 1 2 2 2
  spline S213 degree 2 poles (5.5477, 95.5994) (5.6547, 95.3142) (6.0514, 95.0067) (6.3723, 95.0067) knots 0 0 0 1 2 2 2
  spline S214 degree 2 poles (6.3723, 95.0067) (6.6753, 95.0067) (7.072, 95.2964) (7.1834, 95.5861) knots 0 0 0 1 2 2 2
  line L165 (4.0323, 89.2007) -> (1.6522, 84.5253)
  line L166 (1.6522, 84.5253) -> (0.8678, 84.5253)
  line L167 (0.8678, 84.5253) -> (3.3816, 89.379)
  line L168 (3.3816, 89.379) -> (0.5424, 89.379)
  line L169 (0.5424, 89.379) -> (0.5424, 90.0253)
  line L170 (0.5424, 90.0253) -> (4.0323, 90.0253)
  line L171 (4.0323, 90.0253) -> (4.0323, 89.2007)
  spline S215 degree 2 poles (8.1283, 87.2753) (8.1283, 85.7956) (7.2681, 84.4094) (6.3723, 84.4094) knots 0 0 0 1 2 2 2
  spline S216 degree 2 poles (6.3723, 84.4094) (5.463, 84.4094) (4.6117, 85.8223) (4.6117, 87.2708) knots 0 0 0 1 2 2 2
  spline S217 degree 2 poles (4.6117, 87.2708) (4.6117, 88.7595) (5.4719, 90.1367) (6.3723, 90.1367) knots 0 0 0 1 2 2 2
  spline S218 degree 2 poles (6.3723, 90.1367) (7.277, 90.1367) (8.1283, 88.7105) (8.1283, 87.2753) knots 0 0 0 1 2 2 2
  spline S219 degree 2 poles (7.1834, 85.5994) (7.2904, 85.8713) (7.3796, 86.7093) (7.3796, 87.2753) knots 0 0 0 1 2 2 2
  spline S220 degree 2 poles (7.3796, 87.2753) (7.3796, 87.8413) (7.2904, 88.6748) (7.179, 88.9556) knots 0 0 0 1 2 2 2
  spline S221 degree 2 poles (7.179, 88.9556) (7.0676, 89.2364) (6.6798, 89.5261) (6.3723, 89.5261) knots 0 0 0 1 2 2 2
  spline S222 degree 2 poles (6.3723, 89.5261) (6.0647, 89.5261) (5.6681, 89.2364) (5.5522, 88.9467) knots 0 0 0 1 2 2 2
  spline S223 degree 2 poles (5.5522, 88.9467) (5.4407, 88.6659) (5.3605, 87.8101) (5.3605, 87.2708) knots 0 0 0 1 2 2 2
  spline S224 degree 2 poles (5.3605, 87.2708) (5.3605, 86.6914) (5.4318, 85.9159) (5.5477, 85.6128) knots 0 0 0 1 2 2 2
  spline S225 degree 2 poles (5.5477, 85.6128) (5.6547, 85.3276) (6.0514, 85.02) (6.3723, 85.02) knots 0 0 0 1 2 2 2
  spline S226 degree 2 poles (6.3723, 85.02) (6.6753, 85.02) (7.072, 85.3097) (7.1834, 85.5994) knots 0 0 0 1 2 2 2
  spline S227 degree 2 poles (4.0546, 76.3081) (4.0546, 75.8847) (3.7738, 75.1671) (3.5376, 74.9264) knots 0 0 0 1 2 2 2
  spline S228 degree 2 poles (3.5376, 74.9264) (3.2924, 74.6724) (2.6774, 74.4094) (2.3074, 74.4094) knots 0 0 0 1 2 2 2
  spline S229 degree 2 poles (2.3074, 74.4094) (1.9375, 74.4094) (1.3269, 74.659) (1.0951, 74.9086) knots 0 0 0 1 2 2 2
  spline S230 degree 2 poles (1.0951, 74.9086) (0.8099, 75.2072) (0.489, 76.2101) (0.489, 76.941) knots 0 0 0 1 2 2 2
  spline S231 degree 2 poles (0.489, 76.941) (0.489, 77.6586) (0.7831, 78.813) (1.0907, 79.2409) knots 0 0 0 1 2 2 2
  spline S232 degree 2 poles (1.0907, 79.2409) (1.3893, 79.6598) (2.3342, 80.1278) (2.9537, 80.1278) knots 0 0 0 1 2 2 2
  spline S233 degree 2 poles (2.9537, 80.1278) (3.1364, 80.1278) (3.4574, 80.0922) (3.5777, 80.052) knots 0 0 0 1 2 2 2
  line L172 (3.5777, 80.052) -> (3.5777, 79.3434)
  line L173 (3.5777, 79.3434) -> (3.5465, 79.3434)
  spline S234 degree 2 poles (3.5465, 79.3434) (3.444, 79.3969) (3.0696, 79.4905) (2.8557, 79.4905) knots 0 0 0 1 2 2 2
  spline S235 degree 2 poles (2.8557, 79.4905) (2.1693, 79.4905) (1.3269, 78.5634) (1.2467, 77.6541) knots 0 0 0 1 2 2 2
  spline S236 degree 2 poles (1.2467, 77.6541) (1.5096, 77.8369) (2.0623, 78.0375) (2.3921, 78.0375) knots 0 0 0 1 2 2 2
  spline S237 degree 2 poles (2.3921, 78.0375) (2.713, 78.0375) (3.1944, 77.9082) (3.4574, 77.7121) knots 0 0 0 1 2 2 2
  spline S238 degree 2 poles (3.4574, 77.7121) (3.7604, 77.4848) (4.0546, 76.7806) (4.0546, 76.3081) knots 0 0 0 1 2 2 2
  spline S239 degree 2 poles (3.3058, 76.2769) (3.3058, 76.6157) (3.1275, 77.0747) (2.9314, 77.2352) knots 0 0 0 1 2 2 2
  spline S240 degree 2 poles (2.9314, 77.2352) (2.7843, 77.3511) (2.4189, 77.4268) (2.2272, 77.4268) knots 0 0 0 1 2 2 2
  spline S241 degree 2 poles (2.2272, 77.4268) (1.9687, 77.4268) (1.4829, 77.2708) (1.2467, 77.1238) knots 0 0 0 1 2 2 2
  spline S242 degree 2 poles (1.2467, 77.1238) (1.2422, 77.0435) (1.2333, 76.892) (1.2333, 76.7761) knots 0 0 0 1 2 2 2
  spline S243 degree 2 poles (1.2333, 76.7761) (1.2333, 76.2056) (1.4561, 75.5058) (1.6255, 75.3231) knots 0 0 0 1 2 2 2
  spline S244 degree 2 poles (1.6255, 75.3231) (1.7815, 75.1493) (2.1202, 75.0111) (2.3119, 75.0111) knots 0 0 0 1 2 2 2
  spline S245 degree 2 poles (2.3119, 75.0111) (2.7576, 75.0111) (3.3058, 75.644) (3.3058, 76.2769) knots 0 0 0 1 2 2 2
  spline S246 degree 2 poles (8.1283, 77.2753) (8.1283, 75.7956) (7.2681, 74.4094) (6.3723, 74.4094) knots 0 0 0 1 2 2 2
  spline S247 degree 2 poles (6.3723, 74.4094) (5.463, 74.4094) (4.6117, 75.8223) (4.6117, 77.2708) knots 0 0 0 1 2 2 2
  spline S248 degree 2 poles (4.6117, 77.2708) (4.6117, 78.7595) (5.4719, 80.1367) (6.3723, 80.1367) knots 0 0 0 1 2 2 2
  spline S249 degree 2 poles (6.3723, 80.1367) (7.277, 80.1367) (8.1283, 78.7105) (8.1283, 77.2753) knots 0 0 0 1 2 2 2
  spline S250 degree 2 poles (7.1834, 75.5994) (7.2904, 75.8713) (7.3796, 76.7093) (7.3796, 77.2753) knots 0 0 0 1 2 2 2
  spline S251 degree 2 poles (7.3796, 77.2753) (7.3796, 77.8413) (7.2904, 78.6748) (7.179, 78.9556) knots 0 0 0 1 2 2 2
  spline S252 degree 2 poles (7.179, 78.9556) (7.0676, 79.2364) (6.6798, 79.5261) (6.3723, 79.5261) knots 0 0 0 1 2 2 2
  spline S253 degree 2 poles (6.3723, 79.5261) (6.0647, 79.5261) (5.6681, 79.2364) (5.5522, 78.9467) knots 0 0 0 1 2 2 2
  spline S254 degree 2 poles (5.5522, 78.9467) (5.4407, 78.6659) (5.3605, 77.8101) (5.3605, 77.2708) knots 0 0 0 1 2 2 2
  spline S255 degree 2 poles (5.3605, 77.2708) (5.3605, 76.6914) (5.4318, 75.9159) (5.5477, 75.6128) knots 0 0 0 1 2 2 2
  spline S256 degree 2 poles (5.5477, 75.6128) (5.6547, 75.3276) (6.0514, 75.02) (6.3723, 75.02) knots 0 0 0 1 2 2 2
  spline S257 degree 2 poles (6.3723, 75.02) (6.6753, 75.02) (7.072, 75.3097) (7.1834, 75.5994) knots 0 0 0 1 2 2 2
  spline S258 degree 2 poles (3.912, 66.2725) (3.912, 65.8758) (3.6579, 65.1983) (3.4262, 64.9487) knots 0 0 0 1 2 2 2
  spline S259 degree 2 poles (3.4262, 64.9487) (3.1944, 64.6991) (2.5035, 64.4094) (2.0757, 64.4094) knots 0 0 0 1 2 2 2
  spline S260 degree 2 poles (2.0757, 64.4094) (1.6834, 64.4094) (0.9168, 64.5832) (0.636, 64.7214) knots 0 0 0 1 2 2 2
  line L174 (0.636, 64.7214) -> (0.636, 65.5014)
  line L175 (0.636, 65.5014) -> (0.6895, 65.5014)
  spline S261 degree 2 poles (0.6895, 65.5014) (0.7742, 65.439) (1.0907, 65.2785) (1.2823, 65.2072) knots 0 0 0 1 2 2 2
  spline S262 degree 2 poles (1.2823, 65.2072) (1.5007, 65.1315) (1.8617, 65.0468) (2.089, 65.0468) knots 0 0 0 1 2 2 2
  spline S263 degree 2 poles (2.089, 65.0468) (2.3119, 65.0468) (2.7309, 65.2072) (2.8824, 65.3811) knots 0 0 0 1 2 2 2
  spline S264 degree 2 poles (2.8824, 65.3811) (3.0206, 65.546) (3.1632, 65.9828) (3.1632, 66.2769) knots 0 0 0 1 2 2 2
  spline S265 degree 2 poles (3.1632, 66.2769) (3.1632, 66.5711) (3.0027, 66.9455) (2.8512, 67.0703) knots 0 0 0 1 2 2 2
  spline S266 degree 2 poles (2.8512, 67.0703) (2.6952, 67.2084) (2.2317, 67.3243) (1.9509, 67.3243) knots 0 0 0 1 2 2 2
  spline S267 degree 2 poles (1.9509, 67.3243) (1.6478, 67.3243) (1.0461, 67.2307) (0.8634, 67.1906) knots 0 0 0 1 2 2 2
  line L176 (0.8634, 67.1906) -> (0.8634, 70.0253)
  line L177 (0.8634, 70.0253) -> (3.8808, 70.0253)
  line L178 (3.8808, 70.0253) -> (3.8808, 69.379)
  line L179 (3.8808, 69.379) -> (1.572, 69.379)
  line L180 (1.572, 69.379) -> (1.572, 67.9127)
  spline S268 degree 2 poles (1.572, 67.9127) (1.7057, 67.9305) (1.9642, 67.9439) (2.0712, 67.9439) knots 0 0 0 1 2 2 2
  spline S269 degree 2 poles (2.0712, 67.9439) (2.4946, 67.9439) (3.0785, 67.8057) (3.3459, 67.6007) knots 0 0 0 1 2 2 2
  spline S270 degree 2 poles (3.3459, 67.6007) (3.6178, 67.3956) (3.912, 66.7717) (3.912, 66.2725) knots 0 0 0 1 2 2 2
  spline S271 degree 2 poles (8.1283, 67.2753) (8.1283, 65.7956) (7.2681, 64.4094) (6.3723, 64.4094) knots 0 0 0 1 2 2 2
  spline S272 degree 2 poles (6.3723, 64.4094) (5.463, 64.4094) (4.6117, 65.8223) (4.6117, 67.2708) knots 0 0 0 1 2 2 2
  spline S273 degree 2 poles (4.6117, 67.2708) (4.6117, 68.7595) (5.4719, 70.1367) (6.3723, 70.1367) knots 0 0 0 1 2 2 2
  spline S274 degree 2 poles (6.3723, 70.1367) (7.277, 70.1367) (8.1283, 68.7105) (8.1283, 67.2753) knots 0 0 0 1 2 2 2
  spline S275 degree 2 poles (7.1834, 65.5994) (7.2904, 65.8713) (7.3796, 66.7093) (7.3796, 67.2753) knots 0 0 0 1 2 2 2
  spline S276 degree 2 poles (7.3796, 67.2753) (7.3796, 67.8413) (7.2904, 68.6748) (7.179, 68.9556) knots 0 0 0 1 2 2 2
  spline S277 degree 2 poles (7.179, 68.9556) (7.0676, 69.2364) (6.6798, 69.5261) (6.3723, 69.5261) knots 0 0 0 1 2 2 2
  spline S278 degree 2 poles (6.3723, 69.5261) (6.0647, 69.5261) (5.6681, 69.2364) (5.5522, 68.9467) knots 0 0 0 1 2 2 2
  spline S279 degree 2 poles (5.5522, 68.9467) (5.4407, 68.6659) (5.3605, 67.8101) (5.3605, 67.2708) knots 0 0 0 1 2 2 2
  spline S280 degree 2 poles (5.3605, 67.2708) (5.3605, 66.6914) (5.4318, 65.9159) (5.5477, 65.6128) knots 0 0 0 1 2 2 2
  spline S281 degree 2 poles (5.5477, 65.6128) (5.6547, 65.3276) (6.0514, 65.02) (6.3723, 65.02) knots 0 0 0 1 2 2 2
  spline S282 degree 2 poles (6.3723, 65.02) (6.6753, 65.02) (7.072, 65.3097) (7.1834, 65.5994) knots 0 0 0 1 2 2 2
  line L181 (4.0677, 56.76) -> (3.4126, 56.76)
  line L182 (3.4126, 56.76) -> (3.4126, 54.8703)
  line L183 (3.4126, 54.8703) -> (2.7039, 54.8703)
  line L184 (2.7039, 54.8703) -> (2.7039, 56.76)
  line L185 (2.7039, 56.76) -> (0.2748, 56.76)
  line L186 (0.2748, 56.76) -> (0.2748, 57.5356)
  line L187 (0.2748, 57.5356) -> (2.7351, 60.3703)
  line L188 (2.7351, 60.3703) -> (3.4126, 60.3703)
  line L189 (3.4126, 60.3703) -> (3.4126, 57.3528)
  line L190 (3.4126, 57.3528) -> (4.0677, 57.3528)
  line L191 (4.0677, 57.3528) -> (4.0677, 56.76)
  line L192 (2.7039, 57.3528) -> (2.7039, 59.5011)
  line L193 (2.7039, 59.5011) -> (0.8542, 57.3528)
  line L194 (0.8542, 57.3528) -> (2.7039, 57.3528)
  spline S283 degree 2 poles (8.0791, 57.6203) (8.0791, 56.1405) (7.2189, 54.7544) (6.323, 54.7544) knots 0 0 0 1 2 2 2
  spline S284 degree 2 poles (6.323, 54.7544) (5.4138, 54.7544) (4.5625, 56.1673) (4.5625, 57.6158) knots 0 0 0 1 2 2 2
  spline S285 degree 2 poles (4.5625, 57.6158) (4.5625, 59.1045) (5.4227, 60.4817) (6.323, 60.4817) knots 0 0 0 1 2 2 2
  spline S286 degree 2 poles (6.323, 60.4817) (7.2278, 60.4817) (8.0791, 59.0554) (8.0791, 57.6203) knots 0 0 0 1 2 2 2
  spline S287 degree 2 poles (7.1342, 55.9444) (7.2412, 56.2163) (7.3303, 57.0542) (7.3303, 57.6203) knots 0 0 0 1 2 2 2
  spline S288 degree 2 poles (7.3303, 57.6203) (7.3303, 58.1863) (7.2412, 59.0198) (7.1297, 59.3006) knots 0 0 0 1 2 2 2
  spline S289 degree 2 poles (7.1297, 59.3006) (7.0183, 59.5814) (6.6305, 59.8711) (6.323, 59.8711) knots 0 0 0 1 2 2 2
  spline S290 degree 2 poles (6.323, 59.8711) (6.0155, 59.8711) (5.6188, 59.5814) (5.5029, 59.2916) knots 0 0 0 1 2 2 2
  spline S291 degree 2 poles (5.5029, 59.2916) (5.3915, 59.0109) (5.3113, 58.1551) (5.3113, 57.6158) knots 0 0 0 1 2 2 2
  spline S292 degree 2 poles (5.3113, 57.6158) (5.3113, 57.0364) (5.3826, 56.2609) (5.4984, 55.9578) knots 0 0 0 1 2 2 2
  spline S293 degree 2 poles (5.4984, 55.9578) (5.6054, 55.6725) (6.0021, 55.365) (6.323, 55.365) knots 0 0 0 1 2 2 2
  spline S294 degree 2 poles (6.323, 55.365) (6.6261, 55.365) (7.0228, 55.6547) (7.1342, 55.9444) knots 0 0 0 1 2 2 2
  spline S295 degree 2 poles (2.3776, 49.2493) (2.177, 49.2493) (1.7803, 49.1513) (1.5887, 49.0755) knots 0 0 0 1 2 2 2
  spline S296 degree 2 poles (1.5887, 49.0755) (1.4104, 48.9998) (1.1474, 48.8393) (1.0449, 48.768) knots 0 0 0 1 2 2 2
  line L195 (1.0449, 48.768) -> (1.0004, 48.768)
  line L196 (1.0004, 48.768) -> (1.0004, 49.548)
  spline S297 degree 2 poles (1.0004, 49.548) (1.241, 49.6772) (2.0656, 49.8867) (2.4355, 49.8867) knots 0 0 0 1 2 2 2
  spline S298 degree 2 poles (2.4355, 49.8867) (2.8099, 49.8867) (3.3671, 49.7352) (3.5944, 49.5747) knots 0 0 0 1 2 2 2
  spline S299 degree 2 poles (3.5944, 49.5747) (3.835, 49.4009) (4.0846, 48.8972) (4.0846, 48.5585) knots 0 0 0 1 2 2 2
  spline S300 degree 2 poles (4.0846, 48.5585) (4.0846, 48.1039) (3.4874, 47.4175) (3.0684, 47.3284) knots 0 0 0 1 2 2 2
  line L197 (3.0684, 47.3284) -> (3.0684, 47.2749)
  spline S301 degree 2 poles (3.0684, 47.2749) (3.2423, 47.2392) (3.6389, 47.0788) (3.8083, 46.9183) knots 0 0 0 1 2 2 2
  spline S302 degree 2 poles (3.8083, 46.9183) (3.9777, 46.7623) (4.1916, 46.2631) (4.1916, 45.9021) knots 0 0 0 1 2 2 2
  spline S303 degree 2 poles (4.1916, 45.9021) (4.1916, 45.5322) (3.9376, 44.9037) (3.7058, 44.663) knots 0 0 0 1 2 2 2
  spline S304 degree 2 poles (3.7058, 44.663) (3.4651, 44.4135) (2.7832, 44.1549) (2.3509, 44.1549) knots 0 0 0 1 2 2 2
  spline S305 degree 2 poles (2.3509, 44.1549) (1.9363, 44.1549) (1.1252, 44.3555) (0.8488, 44.4937) knots 0 0 0 1 2 2 2
  line L198 (0.8488, 44.4937) -> (0.8488, 45.2737)
  line L199 (0.8488, 45.2737) -> (0.9023, 45.2737)
  spline S306 degree 2 poles (0.9023, 45.2737) (1.1341, 45.1043) (1.9185, 44.7923) (2.3063, 44.7923) knots 0 0 0 1 2 2 2
  spline S307 degree 2 poles (2.3063, 44.7923) (2.5336, 44.7923) (2.9882, 44.9349) (3.1397, 45.0998) knots 0 0 0 1 2 2 2
  spline S308 degree 2 poles (3.1397, 45.0998) (3.2868, 45.2647) (3.4428, 45.657) (3.4428, 45.9556) knots 0 0 0 1 2 2 2
  spline S309 degree 2 poles (3.4428, 45.9556) (3.4428, 46.2542) (3.269, 46.642) (3.113, 46.7534) knots 0 0 0 1 2 2 2
  spline S310 degree 2 poles (3.113, 46.7534) (2.957, 46.8648) (2.5336, 46.9495) (2.284, 46.9495) knots 0 0 0 1 2 2 2
  line L200 (2.284, 46.9495) -> (1.972, 46.9495)
  line L201 (1.972, 46.9495) -> (1.972, 47.5601)
  line L202 (1.972, 47.5601) -> (2.2171, 47.5601)
  spline S311 degree 2 poles (2.2171, 47.5601) (2.7119, 47.5601) (3.3359, 48.0326) (3.3359, 48.4827) knots 0 0 0 1 2 2 2
  spline S312 degree 2 poles (3.3359, 48.4827) (3.3359, 48.6922) (3.1754, 48.9908) (3.0462, 49.08) knots 0 0 0 1 2 2 2
  spline S313 degree 2 poles (3.0462, 49.08) (2.908, 49.1736) (2.5692, 49.2493) (2.3776, 49.2493) knots 0 0 0 1 2 2 2
  spline S314 degree 2 poles (8.4436, 47.0208) (8.4436, 45.5411) (7.5834, 44.1549) (6.6876, 44.1549) knots 0 0 0 1 2 2 2